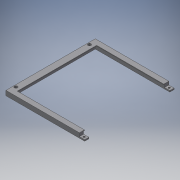
# Autodesk Inventor part: Case-Side
Saved by Autodesk Inventor 2016 SP2 (Build 200236200, 236)
## iProperties
Created: 2018-06-26
Part Number: Case-Side
Material: Generisch
Document SubType Name: Modeling
Designer: Nils
Density: 1 g/cm^3
Appearance: Vorgabe
Author: Nils
Autodesk Inventor part; units mm, degrees
ref_plane "YZ Plane" through (0, 0, 0) normal (1, 0, 0) x (0, 1, 0)
ref_plane "XZ Plane" through (0, 0, 0) normal (0, 1, 0) x (-1, 0, 0)
ref_plane "XY Plane" through (0, 0, 0) normal (0, 0, 1) x (1, 0, 0)
sketch "Skizze1" plane through (0, 0, 0) normal (0, 0, 1) x (1, 0, 0)
  line L0 (0, 0) -> (139.4, 0) construction
  line L1 (139.4, 0) -> (139.4, 169.5) construction
  line L2 (139.4, 169.5) -> (0, 169.5)
  line L3 (0, 169.5) -> (0, 0)
  line L4 (139.4, 160) -> (12, 160)
  line L5 (12, 160) -> (12, 9.5)
  line L6 (12, 9.5) -> (139.4, 9.5)
  line L7 (139.4, 9.5) -> (139.4, 160) construction
  line L8 (0, 0) -> (139.4, 0)
  line L9 (139.4, 0) -> (139.4, 9.5)
  line L10 (139.4, 160) -> (139.4, 169.5)
  dimension "d0" = 9.5
  dimension "d1" = 9.5
  dimension "d2" = 12
  dimension "d3" = 150.5
  dimension "d4" = 127.4
  constraints: 22 end point, 4 parallel, 3 perpendicular, 2 collinear, 2 horizontal, 1 point on line
  measures "d0" distance between parallel lines of L6 L0
  measures "d1" distance between parallel lines of L2 L4
  measures "d2" distance between parallel lines of L5 L3
  measures "d3" distance between parallel lines of L6 L4
  measures "d4" distance of L5.end L6.end
extrude "Extrusion1" add sketch "Skizze1" along normal blind 1.2
sketch "Skizze2" plane through (0, 0, 0) normal (0, 0, -1) x (-1, 0, 0)
  line L0 (-139.4, 8) -> (-8, 8)
  line L1 (-8, 8) -> (-8, 161.5)
  line L2 (-8, 161.5) -> (-139.4, 161.5)
  line L3 (0, 0) -> (-139.4, 0) projected
  line L4 (0, 0) -> (0, 169.5) projected
  line L5 (0, 169.5) -> (-139.4, 169.5) projected
  line L6 (-139.4, 160) -> (-139.4, 169.5) projected
  line L7 (-139.4, 169.5) -> (-149.4, 169.5)
  line L8 (-149.4, 169.5) -> (-149.4, 161.5)
  line L9 (-149.4, 161.5) -> (-139.4, 161.5)
  line L10 (-139.4, 0) -> (-139.4, 9.5) projected
  line L11 (-139.4, 0) -> (-149.4, 0)
  line L12 (-149.4, 0) -> (-149.4, 8)
  line L13 (-149.4, 8) -> (-139.4, 8)
  circle A0 centre (-144.4, 165.5) radius 1.75
  circle A1 centre (-144.4, 4) radius 1.75
  dimension "d7" = 10
  dimension "d8" = 8
  dimension "d9" = 8
  dimension "d10" = 8
  dimension "d11" = 3.5
  dimension "d12" = 5
  dimension "d13" = 4
  dimension "d14" = 3.5
  dimension "d15" = 5
  dimension "d16" = 4
  constraints: 18 end point, 3 perpendicular, 2 centre point, 2 collinear, 2 point on line, 1 horizontal, 1 parallel
  measures "d7" distance of L5.end L7.end
  measures "d8" distance between parallel lines of L3 L0
  measures "d9" distance between parallel lines of L4 L1
  measures "d10" distance between parallel lines of L5 L2
  measures "d11" diameter of A0
  measures "d12" distance from line of L8 A0.centre
  measures "d13" distance from line of L7 A0.centre
  measures "d14" diameter of A1
  measures "d15" distance from line of L12 A1.centre
  measures "d16" distance from line of L13 A1.centre
extrude "Extrusion2" add sketch "Skizze2" along normal blind 7.7
sketch "Skizze3" plane through (0, 0, 0) normal (0, 0, 1) x (1, 0, 0)
  line L0 (139.4, 169.5) -> (139.4, 161.5) projected
  line L1 (139.4, 161.5) -> (149.4, 161.5) projected
  line L2 (149.4, 161.5) -> (149.4, 169.5) projected
  line L3 (149.4, 169.5) -> (139.4, 169.5) projected
  circle A0 centre (144.4, 165.5) radius 1.75 projected
  line L4 (139.4, 8) -> (139.4, 0) projected
  line L5 (139.4, 0) -> (149.4, 0) projected
  line L6 (149.4, 0) -> (149.4, 8) projected
  line L7 (149.4, 8) -> (139.4, 8) projected
  circle A1 centre (144.4, 4) radius 1.75 projected
  point P0 (0, 0)
extrude "Extrusion3" cut sketch "Skizze3" against normal blind 5.1
sketch "Skizze4" plane through (0, 0, 1.2) normal (0, 0, 1) x (1, 0, 0)
  line L0 (139.4, 169.5) -> (0, 169.5) construction
  line L1 (4, 169.5) -> (4, 0) construction
  line L2 (0, 0) -> (139.4, 0) construction
  line L3 (0, 169.5) -> (0, 0) construction
  circle A0 centre (4, 15) radius 3
  circle A1 centre (4, 154.5) radius 3
  dimension "d21" = 4
  dimension "d22" = 6
  dimension "d23" = 6
  dimension "d24" = 15
  dimension "d25" = 15
  constraints: 4 point on line, 2 centre point, 2 end point, 1 vertical
  measures "d21" distance between parallel lines of L3 L1
  measures "d22" diameter of A0
  measures "d23" diameter of A1
  measures "d24" distance from line of L0 A1.centre
  measures "d25" distance from line of L2 A0.centre
extrude "Extrusion4" cut sketch "Skizze4" against normal blind 3.4
sketch "Skizze5" plane through (4, 154.5, -2.2) normal (0, 0, 1) x (1, 0, 0)
  circle A0 centre (0, -139.5) radius 3 projected
  circle A1 centre (0, 0) radius 3 projected
  circle A2 centre (0, 0) radius 3 projected
  circle A3 centre (0, 0) radius 1.75
  circle A4 centre (0, -139.5) radius 1.75
  point P0 (-4, -154.5)
  dimension "d28" = 3.5
  dimension "d29" = 3.5
  constraints: 2 centre point, 2 coincident
  measures "d28" diameter of A3
  measures "d29" diameter of A4
extrude "Extrusion5" cut sketch "Skizze5" against normal blind 42.55 contours A3 | A4
equation "\"d1\" = d0"
equation "\"d14\" = d11"
equation "\"d25\" = d24"
